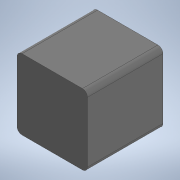
# Autodesk Inventor part: 57 motor
Saved by Autodesk Inventor 2022 (Build 260153000, 153)
## iProperties
Created: 2019-08-15
Part Number: 57 motor
Material: Generic
Document SubType Name: Modeling
Designer: shenglab2
Density: 1 g/cm^3
Appearance: Default
Author: shenglab2
Autodesk Inventor part; units mm, degrees
ref_plane "YZ Plane" through (0, 0, 0) normal (1, 0, 0) x (0, 1, 0)
ref_plane "XZ Plane" through (0, 0, 0) normal (0, 1, 0) x (-1, 0, 0)
ref_plane "XY Plane" through (0, 0, 0) normal (0, 0, 1) x (1, 0, 0)
sketch "Sketch1" plane through (0, 0, 0) normal (0, 0, 1) x (1, 0, 0)
  line L0 (14, -14) -> (-14, -14)
  line L1 (-14, -14) -> (-14, 14)
  line L2 (-14, 14) -> (14, 14)
  line L3 (14, 14) -> (14, -14)
  line L4 (14, -14) -> (-14, 14) construction
  line L5 (-14, -14) -> (14, 14) construction
  point P0 (0, 0)
  dimension "d0" = 28
  dimension "d1" = 28
  constraints: 12 end point, 2 midpoint, 2 parallel, 1 horizontal, 1 perpendicular
  measures "d0" distance of L1.end L2.end
  measures "d1" distance of L0.end L1.end
extrude "Extrusion1" add sketch "Sketch1" along normal blind 30
fillet "Fillet1" radius 2 4 edges at (14, 14, 15) (-14, 14, 15) (14, -14, 15) (-14, -14, 15)
body "Solid1"
